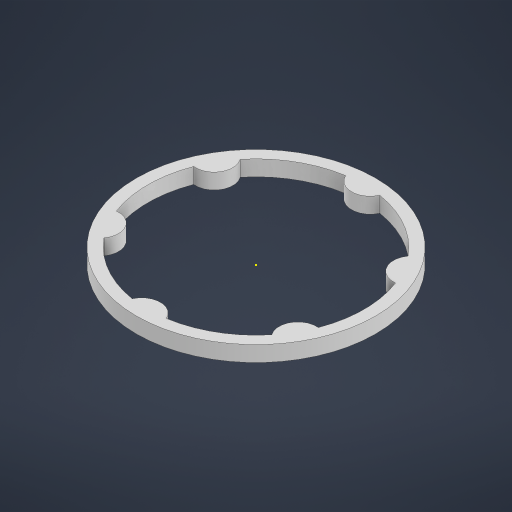
# Autodesk Inventor part: template
Saved by Autodesk Inventor 2024.3 (Build 283343000, 343)
## iProperties
Created: 2025-03-03
Part Number: template
Material: 一般
Document SubType Name: Sheet Metal
Designer: ktamu
Density: 1 g/cm^3
Sheet Metal Rule: Default_mm
Appearance: 既定
Author: ktamu
Autodesk Inventor part; units mm, degrees
ref_plane "YZ Plane" through (0, 0, 0) normal (1, 0, 0) x (0, 1, 0)
ref_plane "XZ Plane" through (0, 0, 0) normal (0, 1, 0) x (-1, 0, 0)
ref_plane "XY Plane" through (0, 0, 0) normal (0, 0, 1) x (1, 0, 0)
sketch "BASEsc" plane through (0, 0, 0) normal (0, 1, 0) x (-1, 0, 0)
  point P0 (0, 0)
sketch "スケッチ2" plane through (0, 0, 0) normal (0, 1, 0) x (-1, 0, 0)
  circle A0 centre (0, 0) radius 17.4
  line L0 (0, -17.4) -> (0, -15.4)
  line L1 (2.75, -16.847) -> (-2.75, -16.847) construction
  line L2 (-2.75, -16.847) -> (-2.75, -17.953) construction
  line L3 (-2.75, -17.953) -> (2.75, -17.953) construction
  line L4 (2.75, -17.953) -> (2.75, -16.847) construction
  line L5 (2.75, -16.847) -> (-2.75, -17.953) construction
  line L6 (-2.75, -16.847) -> (2.75, -17.953) construction
  arc A1 (2.75, -17.1813) -> (-2.75, -17.1813) centre (0, -18.4134) ccw
  arc A2 (16.2545, -6.2091) -> (13.5045, -10.9722) centre (15.9465, -9.2067) ccw
  arc A3 (13.5045, 10.9722) -> (16.2545, 6.2091) centre (15.9465, 9.2067) ccw
  arc A4 (-2.75, 17.1813) -> (2.75, 17.1813) centre (0, 18.4134) ccw
  arc A5 (-16.2545, 6.2091) -> (-13.5045, 10.9722) centre (-15.9465, 9.2067) ccw
  arc A6 (-13.5045, -10.9722) -> (-16.2545, -6.2091) centre (-15.9465, -9.2067) ccw
  circle A7 centre (0, 0) radius 19.25
  point P0 (13.3368, -7.7)
  point P1 (13.3368, 7.7)
  point P2 (0, 15.4)
  point P3 (-13.3368, 7.7)
  point P4 (-13.3368, -7.7)
  point P5 (13.5045, -10.9722)
  point P6 (-13.5045, -10.9722)
  point P7 (-16.2545, -6.2091)
  point P8 (-13.5045, 10.9722)
  point P9 (16.2545, 6.2091)
  dimension "d0" = 34.8
  dimension "d1" = 2
  dimension "d2" = 5.5
  dimension "d5" = 360
  dimension "d7" = 38.5
  constraints: 21 point on circle, 14 end point, 8 centre point, 2 coincident, 2 midpoint, 2 parallel, 2 point on line, 1 horizontal, 1 perpendicular, 1 vertical, 31 other
  measures "d0" diameter of A0
  measures "d1" distance of L0.start L0.end
  measures "d2" distance of L3.end L2.end
  measures "d7" diameter of A7
extrude "押し出し1" add sketch "スケッチ2" along normal blind 2.5 contours A3 A0 | A0 A2 | A4 A0 | A0 L0 A1 | A0 A1 L0 | A5 A0 | A0 A6 | A7
equation "\"BendRadius\" = Thickness"
equation "\"BendReliefWidth\" = Thickness"
equation "\"BendReliefDepth\" = 0.5 * Thickness"
equation "\"CornerReliefSize\" = 4 * Thickness"
equation "\"MinimumRemnant\" = 2 * Thickness"
equation "\"TransitionRadius\" = BendRadius"
equation "\"JacobiRadiusSize\" = BendRadius"
equation "\"GapSize\" = Thickness"
equation "\"Thickness\" = 0.5"
